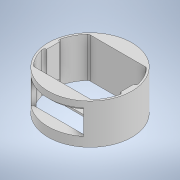
# Autodesk Inventor part: Деталь3
Saved by Autodesk Inventor 2020 (Build 240168000, 168)
## iProperties
Created: 2019-12-15
Part Number: Деталь3
Material: Типовые
Document SubType Name: Modeling
Designer: Валерий
Density: 1 g/cm^3
Appearance: По умолчанию
Author: Валерий
Autodesk Inventor part; units mm, degrees
ref_plane "YZ Plane" through (0, 0, 0) normal (1, 0, 0) x (0, 1, 0)
ref_plane "XZ Plane" through (0, 0, 0) normal (0, 1, 0) x (-1, 0, 0)
ref_plane "XY Plane" through (0, 0, 0) normal (0, 0, 1) x (1, 0, 0)
sketch "Эскиз1" plane through (0, 0, 0) normal (0, 1, 0) x (-1, 0, 0)
  circle A0 centre (0, 0) radius 68
  dimension "d0" = 136
  constraints: 1 centre point, 1 coincident
  measures "d0" diameter of A0
extrude "Выдавливание1" add sketch "Эскиз1" along normal blind 65
sketch "Эскиз2" plane through (0, 0, 0) normal (0, -1, 0) x (1, 0, 0)
  arc A0 (46.7571, -45.1528) -> (64.1997, -10.1682) centre (0, 0) ccw
  line L0 (0, 0) -> (64.1997, -10.1682) construction
  line L1 (0, 0) -> (65, 0) construction
  line L2 (0, 0) -> (46.7571, -45.1528) construction
  arc A1 (-64.1997, -10.1682) -> (-46.7571, -45.1528) centre (0, 0) ccw
  line L3 (0, 0) -> (-64.1997, -10.1682) construction
  line L4 (0, 0) -> (65, 0) construction
  line L5 (0, 0) -> (-46.7571, -45.1528) construction
  line L6 (46.7571, -45.1528) -> (-46.7571, -45.1528)
  line L7 (64.1997, -10.1682) -> (-64.1997, -10.1682)
  dimension "d3" = 65
  dimension "d4" = 9
  dimension "d5" = 35
  dimension "d6" = 65
  dimension "d7" = 171
  dimension "d8" = 35
  constraints: 16 end point, 4 point on circle, 2 centre point, 2 coincident, 2 equal length, 2 horizontal
  measures "d3" radius of A0
  measures "d4" angle of L0 L1
  measures "d5" angle of L2 L0
  measures "d6" radius of A1
  measures "d7" angle of L3 L4
  measures "d8" angle of L3 L5
extrude "Выдавливание2" cut sketch "Эскиз2" against normal blind 65
sketch "Эскиз3" plane through (0, 0, 0) normal (0, -1, 0) x (1, 0, 0)
  arc A0 (64.1997, 10.1682) -> (46.7571, 45.1528) centre (0, 0) ccw
  line L0 (0, 0) -> (64.1997, 10.1682) construction
  line L1 (0, 0) -> (65, 0) construction
  line L2 (0, 0) -> (46.7571, 45.1528) construction
  arc A1 (-46.7571, 45.1528) -> (-64.1997, 10.1682) centre (0, 0) ccw
  line L3 (0, 0) -> (-64.1997, 10.1682) construction
  line L4 (0, 0) -> (65, 0) construction
  line L5 (0, 0) -> (-46.7571, 45.1528) construction
  line L6 (46.7571, 45.1528) -> (-46.7571, 45.1528)
  line L7 (64.1997, 10.1682) -> (-64.1997, 10.1682)
  dimension "d11" = 65
  dimension "d12" = 9
  dimension "d13" = 35
  dimension "d14" = 65
  dimension "d15" = 171
  dimension "d16" = 35
  constraints: 16 end point, 4 point on circle, 2 centre point, 2 coincident, 2 equal length, 2 horizontal
  measures "d11" radius of A0
  measures "d12" angle of L1 L0
  measures "d13" angle of L0 L2
  measures "d14" radius of A1
  measures "d15" angle of L4 L3
  measures "d16" angle of L5 L3
extrude "Выдавливание3" cut sketch "Эскиз3" against normal blind 65
sketch "Эскиз4" plane through (0, 65, 0) normal (0, 1, 0) x (1, 0, 0)
  line L0 (-60, 12.5) -> (60, 12.5)
  line L1 (60, 12.5) -> (60, -12.5)
  line L2 (60, -12.5) -> (-60, -12.5)
  line L3 (-60, -12.5) -> (-60, 12.5)
  line L4 (-60, 12.5) -> (60, -12.5) construction
  line L5 (60, 12.5) -> (-60, -12.5) construction
  point P0 (0, 0)
  dimension "d19" = 120
  dimension "d20" = 25
  constraints: 12 end point, 2 midpoint, 2 parallel, 1 horizontal, 1 perpendicular
  measures "d19" distance of L1.end L2.end
  measures "d20" distance of L0.end L1.end
extrude "Выдавливание4" cut sketch "Эскиз4" against normal blind 62
sketch "Эскиз5" plane through (46.7571, 0, 45.1528) normal (0, 0, -1) x (-1, 0, 0)
  line L0 (89.2571, 15) -> (4.2571, 15)
  line L1 (4.2571, 15) -> (4.2571, 50)
  line L2 (4.2571, 50) -> (89.2571, 50)
  line L3 (89.2571, 50) -> (89.2571, 15)
  line L4 (89.2571, 15) -> (4.2571, 50) construction
  line L5 (4.2571, 15) -> (89.2571, 50) construction
  point P0 (46.7571, 0)
  point P1 (46.7571, 32.5)
  dimension "d23" = 85
  dimension "d24" = 35
  constraints: 12 end point, 2 midpoint, 2 parallel, 1 horizontal, 1 perpendicular
  measures "d23" distance of L1.end L2.end
  measures "d24" distance of L0.end L1.end
extrude "Выдавливание5" cut sketch "Эскиз5" against normal blind 62
chamfer "Фаска1" distance 5 angle 45 1 edges at (0, 15, 45.1528)
chamfer "Фаска2" distance 5 angle 45 1 edges at (0, 50, 68)
fillet "Сопряжение1" radius 10 1 edges at (-60, 3, 0)
fillet "Сопряжение2" radius 10 1 edges at (60, 3, 0)
fillet "Сопряжение3" radius 4 1 edges at (-64.1997, 32.5, 10.1682)
fillet "Сопряжение4" radius 4 1 edges at (-64.1997, 32.5, -10.1682)
fillet "Сопряжение5" radius 4 1 edges at (64.1997, 32.5, -10.1682)
fillet "Сопряжение6" radius 4 1 edges at (64.1997, 32.5, 10.1682)
fillet "Сопряжение7" radius 4 1 edges at (-46.7571, 32.5, -45.1528)
fillet "Сопряжение8" radius 4 1 edges at (46.7571, 32.5, -45.1528)
fillet "Сопряжение9" radius 4 1 edges at (-46.7571, 32.5, 45.1528)
fillet "Сопряжение10" radius 4 1 edges at (46.7571, 32.5, 45.1528)
